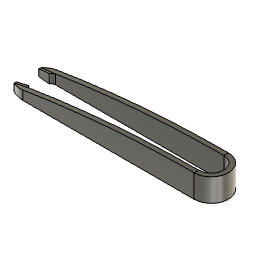
Tweezers v2 (Autodesk Fusion 360 design; units mm, degrees)
Autodesk Fusion 360 part; units mm, degrees
sketch "Sketch1" plane through (0, 0, 0) normal (0, 0, 1) x (1, 0, 0)
  line L0 (-60, 60) -> (50, 80)
  line L1 (50, 80) -> (50, 30)
  line L2 (50, 30) -> (30, 0)
  line L3 (30, 0) -> (-40, 20)
  line L4 (-40, 20) -> (-60, 60)
  constraint vertical L1
sketch "Sketch2" plane through (0, 0, 50) normal (0, 0, 1) x (-1, 0, 0)
  line L0 (40, -20) -> (-30, 0)
  line L1 (-30, 0) -> (-50, -30)
  line L2 (-50, -30) -> (-50, -80)
  line L3 (-50, -80) -> (60, -60)
  line L4 (60, -60) -> (40, -20)
  line L5 (12.353, -51.7329) -> (-20, -51.7329)
  line L6 (-20, -51.7329) -> (-20, -30)
  line L7 (-20, -30) -> (12.353, -30)
  line L8 (12.353, -30) -> (12.353, -51.7329)
  constraint horizontal L5
  constraint vertical L6
  constraint horizontal L7
  constraint vertical L8
sketch "Sketch3" plane through (-12.48, 68.64, 0) normal (-0.178885, 0.98387, 0) x (-0.98387, -0.178885, 0)
  line L0 (-63.5043, 0) -> (48.2991, 0)
  line L1 (48.2991, 0) -> (48.2991, 50)
  line L2 (48.2991, 50) -> (-63.5043, 50)
  line L3 (-63.5043, 50) -> (-63.5043, 0)
  line L4 (-18.8622, 36.1233) -> (0.252, 36.1233)
  line L5 (0.252, 36.1233) -> (0.252, 16.8321)
  line L6 (0.252, 16.8321) -> (-18.8622, 16.8321)
  line L7 (-18.8622, 16.8321) -> (-18.8622, 36.1233)
  constraint horizontal L4
  constraint vertical L5
  constraint horizontal L6
  constraint vertical L7
sketch "Sketch4" plane through (20, 0, 0) normal (1, 0, 0) x (0, 1, 0)
  line L0 (30, 50) -> (51.7329, 50)
  line L1 (51.7329, 50) -> (51.7329, 70)
  line L2 (51.7329, 70) -> (30, 70)
  line L3 (30, 70) -> (30, 50)
  circle A0 centre (40, 60) radius 6.7204
sketch "Sketch5" plane through (0, 0, 0) normal (0, 0, -1) x (1, 0, 0)
sketch "Sketch6" plane through (0, 0, 0) normal (0, 0, 1) x (1, 0, 0)
  line L0 (40, -7.5) -> (-40, -7.5)
  line L1 (-40, 7.5) -> (40, 7.5)
  line L2 (40, -7.5) -> (-40, 7.5) construction
  line L3 (-40, -7.5) -> (40, 7.5) construction
  arc A0 (40, -7.5) -> (40, 7.5) centre (40, 0) ccw
  arc A1 (40, -5.5) -> (40, 5.5) centre (40, 0) ccw
  line L4 (-35, 5.5) -> (40, 5.5)
  line L5 (40, -5.5) -> (-35, -5.5)
  line L6 (-40, -7.5) -> (-40, -5.9374)
  line L7 (-40, 5.9374) -> (-40, 7.5)
  line L8 (-35, 5.5) -> (-40, 5.9374)
  line L9 (-35, -5.5) -> (-40, -5.9374)
  dimension "d11" = 80
  dimension "d12" = 15
  dimension "d15" = 5
  dimension "d17" = 5
  constraint horizontal L0
  constraint perpendicular L0 L6
  constraint parallel L0 L1
  constraint coincident L2 origin
  constraint coincident L3 origin
  constraint tangent L0 A0
  constraint concentric A0 A1
  constraint parallel L1 L4
  constraint parallel L0 L5
  constraint tangent A1 L4
  constraint tangent A1 L5
  constraint collinear L6 L7
  measures "d11" distance of L1.start L1.end
  measures "d12" distance of L0.end L1.start
  measures "d15" angle of L4 L8
  measures "d17" angle of L5 L9
extrude "Extrude6" add sketch "Sketch6" along normal blind 10
sketch "Sketch7" plane through (0, -7.5, 0) normal (0, -1, 0) x (1, 0, 0)
  line L0 (-40, 0) -> (40, 0)
  line L1 (40, 0) -> (40, 10)
  line L2 (40, 10) -> (-40, 10)
  line L3 (-40, 10) -> (-40, 0)
  line L4 (-40, 10) -> (40, 10)
  line L5 (40, 0) -> (40, 10)
  line L6 (40, 0) -> (-40, 0)
  line L7 (-40, 0) -> (-40, 10)
  arc A0 (40, 10) -> (-40, 3) centre (40, -450.6429) ccw
  point P0 (-40, 3)
  dimension "d20" = 3
  constraint coincident L3 P0
  constraint tangent L4 A0
  constraint coincident L1.end L2.start
  constraint coincident P0 A0.end
  measures "d20" distance of L0.start P0
extrude "Extrude7" cut sketch "Sketch7" against normal blind 21 contours L2 L3 L4 L7 A0
extrude "Extrude8" add 1 faces at (-37.5004, 5.7188, 1.1445) along direction (-0.087156, -0.996195, 0) blind 1
extrude "Extrude9" add 1 faces at (-37.5004, -5.7188, 1.1445) along direction (-0.087156, 0.996195, 0) blind 1
fillet "Fillet1" radius 2 1 edges at (-35, 5.5, 1.9267)
fillet "Fillet2" radius 2 1 edges at (-35, -5.5, 1.9267)
fillet "Fillet3" radius 10 1 edges at (-40, 7.5, 1.5)
fillet "Fillet4" radius 10 1 edges at (-40, -7.5, 1.5)
